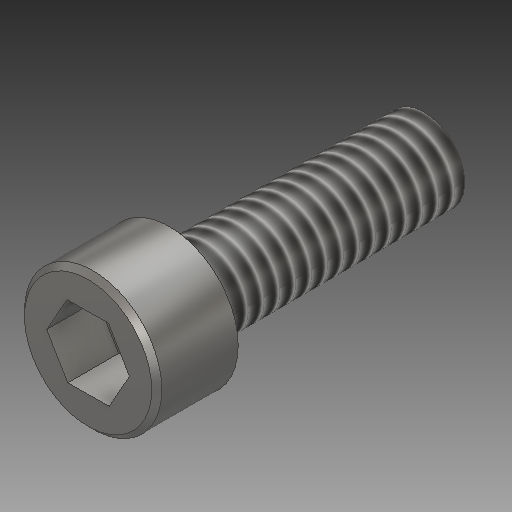
# Autodesk Inventor part: 8-32 UNC Bolt
Saved by Autodesk Inventor 2018 (Build 220112000, 112)
## iProperties
Created: 2018-01-08
Part Number: 8-32 UNC Bolt
Material: Stainless Steel
Document SubType Name: Modeling
Designer: 232963
Density: 8 g/cm^3
Appearance: Semi-Polished
Author: 232963
Autodesk Inventor part; units mm, degrees
ref_plane "YZ Plane" through (0, 0, 0) normal (1, 0, 0) x (0, 1, 0)
ref_plane "XZ Plane" through (0, 0, 0) normal (0, 1, 0) x (-1, 0, 0)
ref_plane "XY Plane" through (0, 0, 0) normal (0, 0, 1) x (1, 0, 0)
sketch "Sketch1" plane through (0, 0, 0) normal (0, 0, 1) x (1, 0, 0)
  circle A0 centre (0, 0) radius 3.429
  dimension "d0" = 6.858
  constraints: 1 centre point, 1 coincident
  measures "d0" diameter of A0
extrude "Extrusion1" add sketch "Sketch1" along normal blind 4.064
sketch "Sketch2" plane through (0, 0, 4.064) normal (0, 0, 1) x (1, 0, 0)
  line L0 (-1.0514, 1.7804) -> (1.0162, 1.8008)
  line L1 (1.0162, 1.8008) -> (2.0676, 0.0204)
  line L2 (2.0676, 0.0204) -> (1.0514, -1.7804)
  line L3 (1.0514, -1.7804) -> (-1.0162, -1.8008)
  line L4 (-1.0162, -1.8008) -> (-2.0676, -0.0204)
  line L5 (-2.0676, -0.0204) -> (-1.0514, 1.7804)
  point P0 (0, 0)
  point P1 (0, 0)
  dimension "d3" = 3.5814
  constraints: 12 end point, 1 coincident, 13 other
  measures "d3" distance between parallel lines of L3 L0
extrude "Extrusion2" cut sketch "Sketch2" against normal blind 2.54
chamfer "Chamfer1" distance 0.254 angle 45 1 edges at (-3.429, 0, 4.064)
sketch "Sketch3" plane through (0, 0, 0) normal (0, 0, -1) x (-1, 0, 0)
  circle A0 centre (0, 0) radius 2.032
  dimension "d9" = 4.064
  constraints: 1 centre point, 1 coincident
  measures "d9" diameter of A0
extrude "Extrusion3" add sketch "Sketch3" along normal blind 12.7
thread "Thread1" size "8-32 UNC" class "2A" standard "ANSI Unified Screw Threads" full length
body "Solid1"
